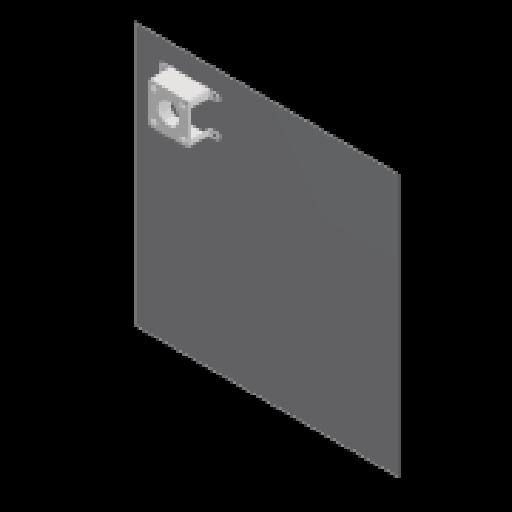
# Autodesk Inventor part: PanpackeMotorMountMK2
Saved by Autodesk Inventor 2025 (Build 290162000, 162)
## iProperties
Created: 2025-01-19
Part Number: PanpackeMotorMountMK2
Material: Generic
Document SubType Name: Modeling
Designer: Trevor
Density: 1 g/cm^3
Appearance: Default
Author: Trevor
Autodesk Inventor part; units mm, degrees
ref_plane "YZ Plane" through (0, 0, 0) normal (1, 0, 0) x (0, 1, 0)
ref_plane "XZ Plane" through (0, 0, 0) normal (0, 1, 0) x (-1, 0, 0)
ref_plane "XY Plane" through (0, 0, 0) normal (0, 0, 1) x (1, 0, 0)
sketch "Sketch1" plane through (0, 0, 0) normal (0, 0, 1) x (1, 0, 0)
  line L0 (-20, 16.5858) -> (-16.5858, 20) projected
  line L1 (-20, -16.5858) -> (-20, 16.5858) projected
  line L2 (-16.5858, -20) -> (-20, -16.5858) projected
  line L3 (16.5858, -20) -> (-16.5858, -20) projected
  line L4 (20, -16.5858) -> (16.5858, -20) projected
  line L5 (20, 16.5858) -> (20, -16.5858) projected
  line L6 (16.5858, 20) -> (20, 16.5858) projected
  line L7 (-16.5858, 20) -> (16.5858, 20) projected
  circle A0 centre (15.5, -15.5) radius 1.5 projected
  circle A1 centre (-15.5, 15.5) radius 1.5 projected
  circle A2 centre (-15.5, -15.5) radius 1.5 projected
  circle A3 centre (15.5, 15.5) radius 1.5 projected
  circle A4 centre (0, 0) radius 11 projected
  line L8 (21, -16.5858) -> (21, 16.5858) projected
  line L9 (-16.5858, -21) -> (16.5858, -21) projected
  line L10 (-21, 16.5858) -> (-21, -16.5858) projected
  line L11 (16.5858, 21) -> (-16.5858, 21) projected
  line L12 (21, 0) -> (21, 21)
  line L13 (21, 21) -> (-21, 21)
  line L14 (-21, 21) -> (-21, 0)
  line L15 (21, 0) -> (21, -21)
  line L16 (21, -21) -> (-21, -21)
  line L17 (-21, -21) -> (-21, 0)
  line L18 (21.5, 21.5) -> (21.5, 0)
  line L19 (21.5, 0) -> (21.5, -21.5)
  line L20 (21.5, -21.5) -> (-21.5, -21.5)
  line L21 (-21.5, -21.5) -> (-21.5, 0)
  line L22 (-21.5, 0) -> (-21.5, 21.5)
  line L23 (-21.5, 21.5) -> (21.5, 21.5)
  dimension "d0" = 0.5
  constraints: 24 end point, 4 parallel, 2 midpoint, 5 other
  measures "d0" distance between parallel lines of L12 L18
ref_plane "Work Plane1" through (-10.7, -10.7, 2) normal (0, 0, 1) x (1, 0, 0)
extrude "Extrusion1" add sketch "Sketch1" along normal up to surface (2 mm away) contours L0 L7 L6 L5 L4 L3 L2 L1 | L15 L16 L9 L17 L10 L14 L13 L11 L12 L8 | L18 L19 L20 L21 L22 L23
ref_plane "Work Plane2" through (-45.7459, -222.85, -21) normal (0, 0, 1) x (1, 0, 0)
sketch "Sketch2" plane through (0, 0, 0) normal (0, 0, -1) x (-1, 0, 0)
  line L0 (-21, 16.5858) -> (-21, 10) projected
  line L1 (-21, 10) -> (-21, -10) projected
  line L2 (-21, -10) -> (-21, -16.5858) projected
  line L3 (21.5, -21.5) -> (-21.5, -21.5) projected
  line L4 (-21.5, 21.5) -> (21.5, 21.5) projected
  line L5 (21.5, 21.5) -> (21.5, -21.5) projected
  line L6 (-21.5, 21.5) -> (21.5, 21.5) projected
  line L7 (-21.5, -21.5) -> (-21.5, 21.5) projected
  line L8 (21.5, -21.5) -> (-21.5, -21.5) projected
  circle A0 centre (0, 0) radius 11 projected
  circle A1 centre (-15.5, 15.5) radius 1.5 projected
  circle A2 centre (15.5, -15.5) radius 1.5 projected
  circle A3 centre (15.5, 15.5) radius 1.5 projected
  circle A4 centre (-15.5, -15.5) radius 1.5 projected
  line L9 (21, -16.5858) -> (21, -10) projected
  line L10 (17.2929, -20.7071) -> (20.7071, -17.2929) projected
  line L11 (20.7071, 17.2929) -> (17.2929, 20.7071) projected
  line L12 (-17.2929, 20.7071) -> (-20.7071, 17.2929) projected
  line L13 (-20.7071, -17.2929) -> (-17.2929, -20.7071) projected
  line L14 (10, -21) -> (16.5858, -21) projected
  line L15 (-16.5858, -21) -> (-10, -21) projected
  arc A5 (20.5642, -14.6074) -> (21.15, -13.1931) centre (19.15, -13.1931) ccw projected
  line L16 (21.15, -13.1931) -> (21.15, 13.1931) projected
  arc A6 (21.15, 13.1931) -> (20.5642, 14.6074) centre (19.15, 13.1931) ccw projected
  line L17 (20.5642, 14.6074) -> (14.6074, 20.5642) projected
  arc A7 (14.6074, 20.5642) -> (13.1931, 21.15) centre (13.1931, 19.15) ccw projected
  line L18 (13.1931, 21.15) -> (-13.1931, 21.15) projected
  arc A8 (-13.1931, 21.15) -> (-14.6074, 20.5642) centre (-13.1931, 19.15) ccw projected
  line L19 (-14.6074, 20.5642) -> (-20.5642, 14.6074) projected
  arc A9 (-20.5642, 14.6074) -> (-21.15, 13.1931) centre (-19.15, 13.1931) ccw projected
  line L20 (-21.15, 13.1931) -> (-21.15, -13.1931) projected
  arc A10 (-21.15, -13.1931) -> (-20.5642, -14.6074) centre (-19.15, -13.1931) ccw projected
  line L21 (-20.5642, -14.6074) -> (-14.6074, -20.5642) projected
  arc A11 (-14.6074, -20.5642) -> (-13.1931, -21.15) centre (-13.1931, -19.15) ccw projected
  line L22 (-13.1931, -21.15) -> (13.1931, -21.15) projected
  arc A12 (13.1931, -21.15) -> (14.6074, -20.5642) centre (13.1931, -19.15) ccw projected
  line L23 (14.6074, -20.5642) -> (20.5642, -14.6074) projected
  circle A13 centre (-15.5, -15.5) radius 1.5 projected
  circle A14 centre (0, 0) radius 4 projected
  circle A15 centre (15.5, -15.5) radius 1.5 projected
  circle A16 centre (15.5, 15.5) radius 1.5 projected
  circle A17 centre (-15.5, 15.5) radius 1.5 projected
  arc A18 (17.2929, 20.7071) -> (16.5858, 21) centre (16.5858, 20) ccw projected
  line L24 (17.2929, 20.7071) -> (20.7071, 17.2929) projected
  arc A19 (21, 16.5858) -> (20.7071, 17.2929) centre (20, 16.5858) ccw projected
  line L25 (21, 16.5858) -> (21, 14.1716) projected
  line L26 (21, 14.1716) -> (14.1716, 21) projected
  line L27 (14.1716, 21) -> (16.5858, 21) projected
  arc A20 (20.7071, -17.2929) -> (21, -16.5858) centre (20, -16.5858) ccw projected
  line L28 (20.7071, -17.2929) -> (17.2929, -20.7071) projected
  arc A21 (16.5858, -21) -> (17.2929, -20.7071) centre (16.5858, -20) ccw projected
  line L29 (16.5858, -21) -> (14.1716, -21) projected
  line L30 (14.1716, -21) -> (21, -14.1716) projected
  line L31 (21, -14.1716) -> (21, -16.5858) projected
  arc A22 (-21, -16.5858) -> (-20.7071, -17.2929) centre (-20, -16.5858) ccw projected
  line L32 (-21, -16.5858) -> (-21, -14.1716) projected
  line L33 (-21, -14.1716) -> (-14.1716, -21) projected
  line L34 (-14.1716, -21) -> (-16.5858, -21) projected
  arc A23 (-17.2929, -20.7071) -> (-16.5858, -21) centre (-16.5858, -20) ccw projected
  line L35 (-17.2929, -20.7071) -> (-20.7071, -17.2929) projected
  arc A24 (-16.5858, 21) -> (-17.2929, 20.7071) centre (-16.5858, 20) ccw projected
  line L36 (-16.5858, 21) -> (-14.1716, 21) projected
  line L37 (-14.1716, 21) -> (-21, 14.1716) projected
  line L38 (-21, 14.1716) -> (-21, 16.5858) projected
  arc A25 (-20.7071, 17.2929) -> (-21, 16.5858) centre (-20, 16.5858) ccw projected
  line L39 (-20.7071, 17.2929) -> (-17.2929, 20.7071) projected
  line L40 (-20.9978, -13.9585) -> (-21.5, -13.9585)
  line L41 (-20.9978, 13.9585) -> (-21.5, 13.9585)
  point P0 (21, -13.9531)
  point P1 (13.9531, -21)
  point P2 (-13.9531, -21)
  point P3 (-21, -13.9531)
  point P4 (-21, 13.9531)
  point P5 (-21, 13.9585)
  point P6 (-21, -13.9585)
  constraints: 4 end point, 2 perpendicular, 2 point on circle, 2 point on line
extrude "Extrusion2" add sketch "Sketch2" along normal up to surface (21 mm away) contours L0 L41 L7 L4 L5 L3 L40 L2 A22 L13 A23 L15 A11 L22 A12 L14 A21 L10 A20 L9 A5 L16 A6 L26 L25 A19 L11 A18 L27 A7 L18 A8 L37 L36 A24 L12 A25
ref_plane "Work Plane3" through (81.2541, -95.85, -21) normal (0, 0, 1) x (0, -1, 0)
sketch "Sketch3" plane through (81.2541, -95.85, -21) normal (0, 0, 1) x (0, -1, 0)
  circle A0 centre (-80.35, -65.7541) radius 1.5 projected
  circle A1 centre (-111.35, -96.7541) radius 1.5 projected
  circle A2 centre (-80.35, -96.7541) radius 1.5 projected
  circle A3 centre (-111.35, -65.7541) radius 1.5 projected
  circle A4 centre (-95.85, -81.2541) radius 11 projected
  line L0 (-117.35, -102.7541) -> (-117.35, -59.7541) projected
  line L1 (-74.35, -102.7541) -> (-117.35, -102.7541) projected
  line L2 (-74.35, -59.7541) -> (-74.35, -102.7541) projected
  line L3 (-117.35, -59.7541) -> (-74.35, -59.7541) projected
  line L4 (-117.35, -102.7541) -> (-74.35, -102.7541)
  line L5 (-74.35, -102.7541) -> (-74.35, -112.7541)
  line L6 (-74.35, -112.7541) -> (-117.35, -112.7541)
  line L7 (-117.35, -112.7541) -> (-117.35, -102.7541)
  circle A5 centre (-95.85, -107.7541) radius 2.5
  line L8 (-117.35, -59.7541) -> (-109.8085, -59.7541) projected
  line L9 (-117.35, -59.7541) -> (-109.8085, -59.7541)
  line L10 (-109.8085, -59.7541) -> (-109.8085, -49.7541)
  line L11 (-109.8085, -49.7541) -> (-117.35, -49.7541)
  line L12 (-117.35, -49.7541) -> (-117.35, -59.7541)
  line L13 (-74.35, -59.7541) -> (-81.85, -59.7541)
  line L14 (-81.85, -59.7541) -> (-81.85, -49.7541)
  line L15 (-81.85, -49.7541) -> (-74.35, -49.7541)
  line L16 (-74.35, -49.7541) -> (-74.35, -59.7541)
  circle A6 centre (-78.1, -54.7541) radius 2.5
  circle A7 centre (-113.5793, -54.7541) radius 2.5
  circle A8 centre (-110.85, -107.7541) radius 2.5
  circle A9 centre (-80.85, -107.7541) radius 2.5
  circle A10 centre (-95.85, -107.7541) radius 2.5
  point P0 (-81.85, -59.7541)
  point P1 (-74.35, -102.7541)
  dimension "d5" = 10
  dimension "d6" = 5
  dimension "d7" = 10
  dimension "d8" = 10
  dimension "d9" = 5
  dimension "d10" = 5
  dimension "d13" = 15
  dimension "d16" = 15
  constraints: 24 end point, 6 centre point, 6 parallel, 5 horizontal, 3 perpendicular, 6 other
  measures "d5" distance of L4.end L5.end
  measures "d6" diameter of A5
  measures "d7" distance of L10.end L9.end
  measures "d8" distance of L13.end L14.end
  measures "d9" diameter of A6
  measures "d10" diameter of A7
  measures "d13" distance of A5.centre A8.centre
  measures "d16" distance of A5.centre A9.centre
extrude "Extrusion3" add sketch "Sketch3" along normal blind 1 contours L1 L5 L6 L7 | L12 L11 L10 L3 | L3 L14 L15 L16
fillet "Fillet1" radius 2 8 edges at (21.5, 21.5, 1) (21.5, 21.5, -10) (21.5, -21.5, 1) (21.5, -21.5, -10) (-21.5, -21.5, -10) (-21.5, -21.5, 1) (-21.5, 21.5, 1) (-21.5, 21.5, -10)
fillet "Fillet2" radius 2 6 edges at (31.5, -21.5, -20.5) (31.5, -14, -20.5) (31.5, 13.9585, -20.5) (31.5, 21.5, -20.5) (-31.5, -21.5, -20.5) (-31.5, 21.5, -20.5)
chamfer "Chamfer1" distance 2 angle 45 4 edges at (14, -15.5, 2) (14, 15.5, 2) (-17, 15.5, 2) (-17, -15.5, 2)
body "Solid1"
